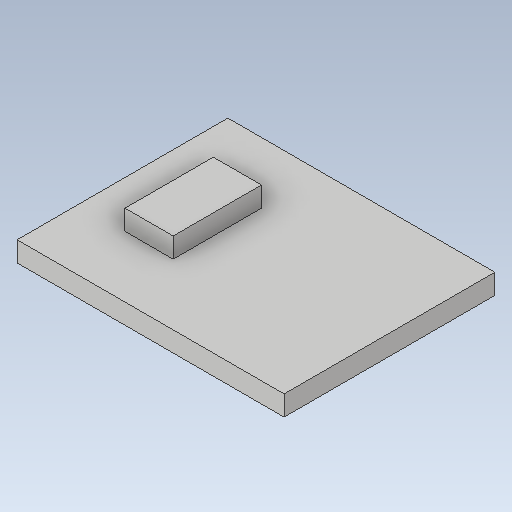
# Autodesk Inventor part: vl
Saved by Autodesk Inventor 2020 (Build 240168000, 168)
## iProperties
Created: 2019-02-22
Part Number: vl
Material: Ogólny
Document SubType Name: Modeling
Designer: atmat
Density: 1 g/cm^3
Appearance: Domyślna
Author: atmat
Autodesk Inventor part; units mm, degrees
ref_plane "YZ Plane" through (0, 0, 0) normal (1, 0, 0) x (0, 1, 0)
ref_plane "XZ Plane" through (0, 0, 0) normal (0, 1, 0) x (-1, 0, 0)
ref_plane "XY Plane" through (0, 0, 0) normal (0, 0, 1) x (1, 0, 0)
sketch "Szkic1" plane through (0, 0, 0) normal (0, 1, 0) x (-1, 0, 0)
  line L0 (6.65, 5.25) -> (-6.65, 5.25)
  line L1 (-6.65, 5.25) -> (-6.65, -5.25)
  line L2 (-6.65, -5.25) -> (6.65, -5.25)
  line L3 (6.65, -5.25) -> (6.65, 5.25)
  point P0 (0, 0)
  dimension "d0" = 10.5
  dimension "d1" = 5.25
  dimension "d2" = 6.65
  dimension "d3" = 13.3
  constraints: 8 end point, 2 parallel, 1 horizontal, 1 perpendicular
  measures "d0" distance of L2.end L0.start
  measures "d1" distance from line of point (0, 0) L0
  measures "d2" distance from line of point (0, 0) L1
  measures "d3" distance of L1.end L2.end
extrude "Wyciągnięcie proste1" add sketch "Szkic1" along normal blind 1
sketch "Szkic2" plane through (0, 1, 0) normal (0, 1, 0) x (1, 0, 0)
  line L0 (-4.3267, -2.2) -> (-1.9267, -2.2)
  line L1 (-1.9267, -2.2) -> (-1.9267, 2.2)
  line L2 (-1.9267, 2.2) -> (-4.3267, 2.2)
  line L3 (-4.3267, 2.2) -> (-4.3267, -2.2)
  point P0 (0, 0)
  dimension "d6" = 4.4
  dimension "d7" = 2.4
  dimension "d8" = 2.2
  constraints: 8 end point, 2 parallel, 1 horizontal, 1 perpendicular
  measures "d6" distance of L2.end L0.start
  measures "d7" distance of L1.end L2.end
  measures "d8" distance from line of point (0, 0) L2
extrude "Wyciągnięcie proste2" add sketch "Szkic2" along normal blind 1
